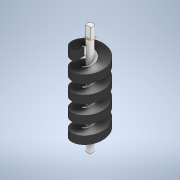
# Autodesk Inventor part: Tornillo
Saved by Autodesk Inventor 2020.3 (Build 243373000, 373)
## iProperties
Created: 2020-08-17
Part Number: Tornillo
Material: ABS Plastic
Document SubType Name: Modeling
Designer: juanp
Density: 1.06 g/cm^3
Appearance: Smooth - White
Author: juanp
Autodesk Inventor part; units mm, degrees
ref_plane "YZ Plane" through (0, 0, 0) normal (1, 0, 0) x (0, 1, 0)
ref_plane "XZ Plane" through (0, 0, 0) normal (0, 1, 0) x (-1, 0, 0)
ref_plane "XY Plane" through (0, 0, 0) normal (0, 0, 1) x (1, 0, 0)
sketch "Sketch1" plane through (0, 0, 0) normal (0, 1, 0) x (-1, 0, 0)
  circle A0 centre (0, 0) radius 2.5
  dimension "d0" = 5
  constraints: 1 centre point, 1 coincident
  measures "d0" diameter of A0
extrude "Extrusion1" add sketch "Sketch1" along normal blind 72
sketch "Sketch2" plane through (0, 0, 0) normal (1, 0, 0) x (0, 1, 0)
  line L0 (0, -2.5) -> (0, 2.5) projected
  line L1 (0, -2.5) -> (6.4, -2.5)
  line L2 (6.4, -2.5) -> (6.4, -4.7)
  line L3 (6.4, -4.7) -> (0, -4.7)
  line L4 (0, -4.7) -> (0, -2.5)
  point P0 (0, 0)
  dimension "d3" = 6.4
  dimension "d4" = 2.2
  constraints: 8 end point, 2 parallel, 1 horizontal, 1 perpendicular
  measures "d3" distance of L2.end L3.end
  measures "d4" distance of L1.end L2.end
coil "Coil1" sketch "Sketch2" operation add axis through (0, 0, 0) along (0, 1, 0) pitch 14.4444 turns 4.5 hand right
sketch "Sketch3" plane through (0, 65, 2.5) normal (1, 0, 0) x (0, 0, -1)
  line L0 (-2.2, 6.4) -> (-2.2, 0) projected
  line L1 (-2.2, 6.4) -> (-10.2, 6.4)
  line L2 (-10.2, 6.4) -> (-10.2, 0)
  line L3 (-10.2, 0) -> (-2.2, 0)
  line L4 (-2.2, 0) -> (-2.2, 6.4)
  point P0 (2.5, -65)
  dimension "d14" = 8
  constraints: 8 end point, 2 parallel, 1 horizontal, 1 perpendicular
  measures "d14" distance between parallel lines of L0 L2
coil "Coil2" sketch "Sketch3" operation add axis through (0, 0, 0) along (0, -1, 0) pitch 14.4444 turns 4.5 hand right separate body
sketch "Sketch8" plane through (0, 0, 0) normal (0, -1, 0) x (1, 0, 0)
  circle A0 centre (0, 0) radius 2.5
  dimension "d32" = 5
  constraints: 1 centre point, 1 coincident
  measures "d32" diameter of A0
extrude "Extrusion5" add sketch "Sketch8" along normal blind 4.5 bodies 1
sketch "Sketch9" plane through (0, 72, 0) normal (0, 1, 0) x (1, 0, 0)
  circle A0 centre (0, 0) radius 2.5
  dimension "d35" = 5
  constraints: 1 centre point, 1 coincident
  measures "d35" diameter of A0
extrude "Extrusion6" add sketch "Sketch9" along normal blind 12.67 bodies 1
ref_plane "Work Plane2" through (0, 76, 0) normal (0, 1, 0) x (1, 0, 0)
sketch "Sketch13" plane through (0, 76, 0) normal (0, 1, 0) x (1, 0, 0)
  circle A0 centre (0, 0) radius 2.5 projected
  line L0 (2, -1.5) -> (-2, -1.5)
  dimension "d47" = 1
  constraints: 2 end point, 2 point on circle, 1 horizontal
  measures "d47" distance edge to line of A0 L0
extrude "Extrusion9" cut sketch "Sketch13" along normal through all contours L0 A0 picked at (-0.534, -1.6398) bodies 1
body "Solid1"
body "Solid2"
